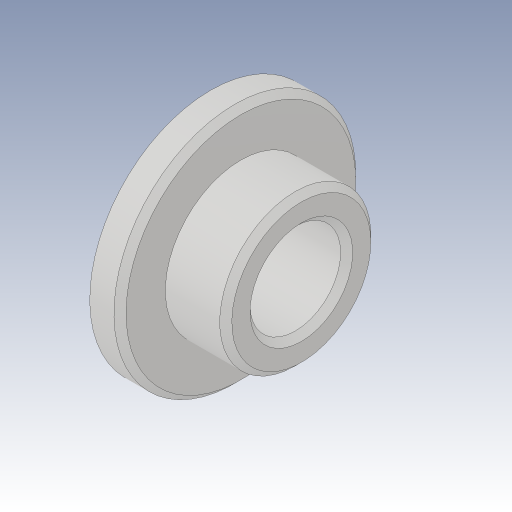
# Autodesk Inventor part: BT014_huenin20_23
Saved by Autodesk Inventor 2023.3 (Build 273359000, 359)
## iProperties
Company: HTBLA Kaindorf
RuleStatus: InUse
Created: 2023-12-01
Part Number: BT014_huenin20_23
Project: Fiberprinter-Hotend
Material: S235JR
Description: Faservorschubgleitlager
Document SubType Name: Modeling
Designer: huenin20
Density: 7.85 g/cm^3
Appearance: Metall
Mass: 0.527016 g
Surface Area: 1.64224 cm^2
Volume: 0.0671358 cm^3
AfterDocNew0: iProperties-Editor_aufrufen
Author: nicob
Keywords: 2023
Autodesk Inventor part; units mm, degrees
ref_plane "YZ Plane" through (0, 0, 0) normal (1, 0, 0) x (0, 1, 0)
ref_plane "XZ Plane" through (0, 0, 0) normal (0, 1, 0) x (-1, 0, 0)
ref_plane "XY Plane" through (0, 0, 0) normal (0, 0, 1) x (1, 0, 0)
sketch "Skizze3" plane through (0, 0, 0) normal (1, 0, 0) x (0, 1, 0)
  line L0 (0, 0) -> (4.4378, 0)
  line L1 (0, 1.5) -> (3, 1.5)
  line L2 (3, 1.5) -> (3, 2.5)
  line L3 (3, 2.5) -> (1, 2.5)
  line L4 (1, 2.5) -> (1, 4)
  line L5 (1, 4) -> (0, 4)
  line L6 (0, 4) -> (0, 1.5)
  dimension "d4" = 1
  dimension "d5" = 3
  dimension "d6" = 3
  dimension "d7" = 8
  dimension "d8" = 5
  constraints: 14 end point, 4 perpendicular, 2 horizontal, 1 parallel, 1 vertical alignment
  measures "d4" distance of L4.end L5.end
  measures "d5" distance of L1.start L1.end
  measures "d6" diameter of L1 L0
  measures "d7" diameter of L5 L0
  measures "d8" diameter of L3 L0
revolve "Umdrehung1" add sketch "Skizze3" angle 360 about axis through (0, 0, 0) along (0, 1, 0)
chamfer "Fase1" distance 0.2 angle 45 4 edges at (0, 3, -2.5) (0, 3, -1.5) (0, 1, -4) (0, 0, -1.5)
